mount to motor plate v1 (Autodesk Fusion 360 design; units mm, degrees)
Autodesk Fusion 360 part; units mm, degrees
sketch "Sketch1" plane through (0, 0, 0) normal (0, 1, 0) x (1, 0, 0)
  line L0 (75, -25) -> (-75, -25)
  line L1 (-75, -25) -> (-75, 25)
  line L2 (-75, 25) -> (75, 25)
  line L3 (75, 25) -> (75, -25)
  line L4 (75, -25) -> (-75, 25) construction
  line L5 (-75, -25) -> (75, 25) construction
  dimension "d1" = 150
  dimension "d2" = 50
  constraint horizontal L0
  constraint perpendicular L0 L1
  constraint parallel L0 L2
  constraint parallel L1 L3
  constraint coincident L4 origin
  constraint coincident L5 origin
  measures "d1" distance of L1.end L2.end
  measures "d2" distance of L0.end L1.end
extrude "Extrude1" add sketch "Sketch1" along normal blind 65
sketch "Sketch2" plane through (0, 0, 25) normal (0, 0, 1) x (1, 0, 0)
  line L0 (-75, 0) -> (75, 0)
  line L1 (75, 0) -> (75, 65)
  line L2 (75, 65) -> (-75, 65)
  line L3 (-75, 65) -> (-75, 0)
  line L4 (-75, 0) -> (75, 0)
  line L5 (75, 0) -> (75, 15)
  line L6 (75, 15) -> (-75, 15)
  line L7 (-75, 15) -> (-75, 0)
  line L8 (-75, 65) -> (-50, 65)
  line L9 (-50, 65) -> (-50, 15)
  line L10 (-50, 15) -> (-75, 15)
  line L11 (-75, 15) -> (-75, 65)
  line L12 (75, 65) -> (50, 65)
  line L13 (50, 65) -> (50, 15)
  line L14 (50, 15) -> (75, 15)
  line L15 (75, 15) -> (75, 65)
  line L16 (-50, 65) -> (-30, 65)
  line L17 (-30, 65) -> (-30, 15)
  line L18 (-30, 15) -> (-50, 15)
  line L19 (-50, 15) -> (-50, 65)
  line L20 (-30, 65) -> (-10, 65)
  line L21 (-10, 65) -> (-10, 15)
  line L22 (-10, 15) -> (-30, 15)
  line L23 (-30, 15) -> (-30, 65)
  line L24 (-10, 65) -> (10, 65)
  line L25 (10, 65) -> (10, 15)
  line L26 (10, 15) -> (-10, 15)
  line L27 (-10, 15) -> (-10, 65)
  line L28 (10, 65) -> (30, 65)
  line L29 (30, 65) -> (30, 15)
  line L30 (30, 15) -> (10, 15)
  line L31 (10, 15) -> (10, 65)
  line L32 (30, 65) -> (50, 65)
  line L33 (50, 65) -> (50, 15)
  line L34 (50, 15) -> (30, 15)
  line L35 (30, 15) -> (30, 65)
  dimension "d5" = 150
  dimension "d6" = 15
  dimension "d7" = 20
  dimension "d8" = 20
  dimension "d9" = 20
  dimension "d10" = 20
  dimension "d11" = 20
  dimension "d12" = 25
  constraint horizontal L4
  constraint vertical L5
  constraint horizontal L6
  constraint vertical L7
  constraint coincident L0.start L3.end
  constraint horizontal L8
  constraint vertical L9
  constraint horizontal L10
  constraint vertical L11
  constraint coincident L6 L9.end
  constraint coincident L2.end L3.start
  constraint horizontal L12
  constraint vertical L13
  constraint horizontal L14
  constraint vertical L15
  constraint coincident L6 L13.end
  constraint coincident L1.end L2.start
  constraint horizontal L16
  constraint vertical L17
  constraint horizontal L18
  constraint vertical L19
  constraint coincident L6 L17.end
  constraint horizontal L20
  constraint vertical L21
  constraint horizontal L22
  constraint vertical L23
  constraint coincident L6 L21.end
  constraint horizontal L24
  constraint vertical L25
  constraint horizontal L26
  constraint vertical L27
  constraint coincident L6 L25.end
  constraint horizontal L28
  constraint vertical L29
  constraint horizontal L30
  constraint vertical L31
  constraint coincident L6 L29.end
  constraint horizontal L32
  constraint vertical L33
  constraint horizontal L34
  constraint vertical L35
  measures "d5" distance of L0.start L0.end
  measures "d6" distance of L0.start L6.end
  measures "d7" distance of L9 L17
  measures "d8" distance of L21 L23
  measures "d9" distance of L27 L31
  measures "d10" distance of L25 L35
  measures "d11" distance of L29 L33
  measures "d12" distance of L11 L19
extrude "Extrude2" cut sketch "Sketch2" against normal blind 50 contours L2 L6 L9 L16 L17 L18 L19 L23 | L2 L6 L13 L29 L32 L33 L34 L35 | L2 L6 L21 L24 L25 L26 L27 L31
sketch "Sketch3" plane through (-75, 0, 0) normal (-1, 0, 0) x (0, 0, 1)
  line L0 (-25, 0) -> (25, 0)
  line L1 (25, 0) -> (25, 65)
  line L2 (25, 65) -> (-25, 65)
  line L3 (-25, 65) -> (-25, 0)
  circle A0 centre (0, 40) radius 25
  dimension "d15" = 40
  constraint tangent L2 A0
  measures "d15" distance of origin A0.centre
extrude "Extrude3" cut sketch "Sketch3" against normal blind 150 contours L2 L3 A0 | L1 L2 A0
sketch "Sketch4" plane through (0, 15, 0) normal (0, 1, 0) x (-1, 0, 0)
  line L0 (50, 25) -> (30, 25)
  line L1 (30, 25) -> (30, -25)
  line L2 (30, -25) -> (50, -25)
  line L3 (50, -25) -> (50, 25)
  circle A0 centre (40, 0) radius 5
  circle A1 centre (0, 0) radius 5
  circle A2 centre (-40, 0) radius 5
  constraint coincident A1.centre origin
hole "Hole1" at (-40, 15, 0) at (0, 15, 0) at (40, 15, 0) direction (0, -1, 0) diameter 10 depth 30 tip angle 118 counterbore diameter 16 counterbore depth 10
sketch "Sketch5" plane through (-75, 0, 0) normal (-1, 0, 0) x (0, 0, 1)
  arc A0 (25, 40) -> (-25, 40) centre (0, 40) ccw
  line L0 (-25, 40) -> (-25, 0)
  line L1 (-25, 0) -> (25, 0)
  line L2 (25, 0) -> (25, 40)
  circle A1 centre (0, 40) radius 25
  dimension "d23" = 50
  constraint concentric A0 A1
  measures "d23" diameter of A1
hole "Hole2" at (-75, 40, 0) direction (1, 0, 0) diameter 25 depth 150 tip angle 180
